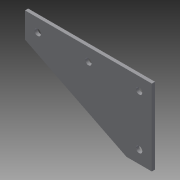
# Autodesk Inventor part: CatapultGussetPlate
Saved by Autodesk Inventor 2013 (Build 170138000, 138)
## iProperties
Created: 2014-01-18
Part Number: CatapultGussetPlate
Material: Generic
Document SubType Name: Modeling
Designer: 215152
Density: 1 g/cm^3
Author: 215152
Autodesk Inventor part; units mm, degrees
ref_plane "YZ Plane" through (0, 0, 0) normal (1, 0, 0) x (0, 1, 0)
ref_plane "XZ Plane" through (0, 0, 0) normal (0, 1, 0) x (-1, 0, 0)
ref_plane "Work Plane1" through (0, 0, 0) normal (0, 0, 1) x (1, 0, 0)
sketch "Sketch1" plane through (0, 0, 0) normal (0, 0, 1) x (1, 0, 0)
  line L0 (0, 0) -> (673.1, 0)
  line L1 (673.1, 0) -> (673.1, -25.4)
  line L2 (673.1, -25.4) -> (0, -25.4)
  line L3 (0, -25.4) -> (0, 0)
  line L4 (673.1, 0) -> (419.1, 0)
  line L5 (419.1, 0) -> (419.1, -25.4)
  line L6 (419.1, -25.4) -> (673.1, -25.4)
  line L7 (673.1, -25.4) -> (673.1, 0)
  line L8 (419.1, 0) -> (393.7, 0)
  line L9 (393.7, -127) -> (419.1, -127)
  line L10 (419.1, -127) -> (419.1, 0)
  line L11 (419.1, 0) -> (292.1, 0)
  line L12 (292.1, 0) -> (292.1, -25.4)
  line L13 (419.1, -25.4) -> (419.1, 0)
  line L14 (393.7, -127) -> (292.1, -25.4)
  line L15 (292.1, -12.7) -> (304.8, -12.7) construction
  line L16 (406.4, -12.7) -> (457.2, -12.7) construction
  circle A0 centre (406.4, -12.7) radius 3.175
  circle A1 centre (406.4, -63.5) radius 3.175
  circle A2 centre (406.4, -114.3) radius 3.175
  circle A3 centre (304.8, -12.7) radius 3.175
  line L17 (406.4, -12.7) -> (457.2, -12.7) construction
  circle A4 centre (355.6, -12.7) radius 3.175
  dimension "d0" = 673.1
  dimension "d1" = 25.4
  dimension "d2" = 254
  dimension "d3" = 25.4
  dimension "d4" = 25.4
  dimension "d5" = 127
  dimension "d6" = 127
  dimension "d7" = 25.4
  dimension "d14" = 6.35
  dimension "d15" = 6.35
  dimension "d16" = 6.35
  dimension "d17" = 6.35
  dimension "d20" = 6.35
  constraints: 36 end point, 7 horizontal, 6 parallel, 5 centre point, 3 perpendicular, 2 coincident, 1 midpoint
  measures "d0" distance of L1.end L2.end
  measures "d1" distance of L0.end L1.end
  measures "d2" distance of L6.end L5.end
  measures "d3" distance of L5.end L4.end
  measures "d4" distance of L9.end L9.start
  measures "d5" distance of L9.start L8.end
  measures "d6" distance of L13.start L12.end
  measures "d7" distance of L12.end L11.end
  measures "d14" diameter of A0
  measures "d15" diameter of A1
  measures "d16" diameter of A2
  measures "d17" diameter of A3
  measures "d20" diameter of A4
extrude "Extrusion1" add sketch "Sketch1" along normal blind 3.175 contours L0 L5 L2 L12 | L2 L10 L9 L14
sketch "Sketch2" plane through (0, 0, 3.175) normal (0, 0, 1) x (1, 0, 0)
  circle A0 centre (406.4, -114.3) radius 3.175 projected
  line L0 (419.1, 0) -> (292.1, 0) projected
  line L1 (292.1, 0) -> (292.1, -25.4) projected
  line L2 (292.1, -25.4) -> (393.7, -127) projected
  line L3 (393.7, -127) -> (419.1, -127) projected
  line L4 (419.1, -127) -> (419.1, 0) projected
  line L5 (419.1, 0) -> (393.7, 0)
  line L6 (393.7, 0) -> (393.7, -76.2)
  line L7 (393.7, -76.2) -> (419.1, -76.2)
  line L8 (419.1, -76.2) -> (419.1, 0)
  line L9 (393.7, -76.2) -> (292.1, -25.4)
  point P0 (0, 0)
  dimension "d23" = 25.4
  dimension "d24" = 76.2
  constraints: 10 end point, 2 parallel, 1 horizontal, 1 perpendicular
  measures "d23" distance of L7.end L6.end
  measures "d24" distance of L6.end L5.end
extrude "Extrusion2" cut sketch "Sketch2" against normal blind 25.4 contours L4 L3 L2 L9 L7
body "Solid1"
